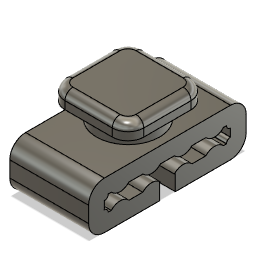
Helmet Mask Holder v3 (Autodesk Fusion 360 design; units mm, degrees)
Autodesk Fusion 360 part; units mm, degrees
sketch "Sketch1" plane through (0, 0, 0) normal (0, 1, 0) x (1, 0, 0)
  line L0 (-2770, 2200) -> (-2760, 2200)
  line L1 (-2760, 2200) -> (-2760, 2180)
  line L2 (-2760, 2180) -> (-2770, 2180)
  line L3 (-2770, 2180) -> (-2770, 2200)
  dimension "d3" = 10
  dimension "d4" = 20
  constraint horizontal L0
  constraint vertical L1
  constraint horizontal L2
  constraint vertical L3
  measures "d3" distance of L0.start L0.end
  measures "d4" distance of L0.start L2.end
extrude "Extrude1" add sketch "Sketch1" along normal blind 6 makes body 1
fillet "Fillet1" radius 2 4 edges at (-2765, 0, -2200) (-2765, 6, -2200) (-2765, 6, -2180) (-2765, 0, -2180) on bodies 1
sketch "Sketch2" plane through (-2760, 0, 0) normal (1, 0, 0) x (0, 0, -1)
  arc A0 (2180, 2) -> (2182, 0) centre (2182, 2) ccw
  line L0 (2182, 0) -> (2198, 0)
  arc A1 (2198, 0) -> (2200, 2) centre (2198, 2) ccw
  line L1 (2200, 2) -> (2200, 4)
  arc A2 (2200, 4) -> (2198, 6) centre (2198, 4) ccw
  line L2 (2198, 6) -> (2182, 6)
  arc A3 (2182, 6) -> (2180, 4) centre (2182, 4) ccw
  line L3 (2180, 4) -> (2180, 2)
  line L4 (2182, 4) -> (2198, 4)
  line L5 (2198, 4) -> (2198, 2)
  line L6 (2198, 2) -> (2182, 2)
  line L7 (2182, 2) -> (2182, 4)
  line L8 (2189.0127, 2) -> (2191, 2)
  line L9 (2191, 2) -> (2191, 0)
  line L10 (2191, 0) -> (2189.0127, 0)
  line L11 (2189.0127, 0) -> (2189.0127, 2)
  circle A4 centre (2184, 5) radius 1.5
  circle A5 centre (2184, 1) radius 1.5
  circle A6 centre (2188, 5) radius 1.5
  circle A7 centre (2188, 1) radius 1.5
  circle A8 centre (2192, 5) radius 1.5
  circle A9 centre (2192, 1) radius 1.5
  circle A10 centre (2196, 5) radius 1.5
  circle A11 centre (2196, 1) radius 1.5
  circle A12 centre (2182, 4) radius 0.5
  circle A13 centre (2182, 2) radius 0.5
  circle A14 centre (2198, 4) radius 0.5
  circle A15 centre (2198, 2) radius 0.5
  dimension "d9" = 3
  dimension "d10" = 3
  dimension "d11" = 3
  dimension "d12" = 3
  dimension "d13" = 3
  dimension "d14" = 3
  dimension "d15" = 3
  dimension "d16" = 3
  dimension "d28" = 1
  dimension "d29" = 1
  dimension "d30" = 1
  dimension "d31" = 1
  constraint horizontal L4
  constraint vertical L5
  constraint horizontal L6
  constraint vertical L7
  constraint coincident A1.centre L5.end
  constraint coincident A3.centre L4.start
  constraint horizontal L8
  constraint vertical L9
  constraint horizontal L10
  constraint vertical L11
  constraint coincident L0 L9.end
  constraint coincident L6 L8.start
  constraint concentric A0 A13
  constraint concentric A2 A14
  measures "d9" diameter of A4
  measures "d10" diameter of A5
  measures "d11" diameter of A6
  measures "d12" diameter of A7
  measures "d13" diameter of A8
  measures "d14" diameter of A9
  measures "d15" diameter of A10
  measures "d16" diameter of A11
  measures "d28" diameter of A12
  measures "d29" diameter of A13
  measures "d30" diameter of A14
  measures "d31" diameter of A15
extrude "Extrude2" cut sketch "Sketch2" against normal blind 30 contours L4 L5 L6 L7 L8 A4 A5 A6 A7 A8 A9 A10 A11 A12 A13 A14 A15 | L0 L6 L8 L10 L11 A7 | L0 L6 L8 L10 A7 A9 | L0 L6 L8 L9 L10 A9 bodies 1
sketch "Sketch3" plane through (0, 6, 0) normal (0, 1, 0) x (-1, 0, 0)
  line L0 (2770, -2182) -> (2760, -2182)
  line L1 (2760, -2182) -> (2760, -2198)
  line L2 (2770, -2198) -> (2770, -2182)
  circle A0 centre (2765, -2190) radius 4
  line L3 (2760, -2198) -> (2770, -2198)
  dimension "d27" = 8
  measures "d27" diameter of A0
extrude "Extrude3" add sketch "Sketch3" along normal blind 2 separate body contours A0 makes body 2
sketch "Sketch4" plane through (0, 8, 0) normal (0, 1, 0) x (-1, 0, 0)
  circle A0 centre (2765, -2190) radius 5
  circle A1 centre (2765, -2190) radius 4
  line L0 (2770, -2195) -> (2760, -2195)
  line L1 (2760, -2195) -> (2760, -2185)
  line L2 (2760, -2185) -> (2770, -2185)
  line L3 (2770, -2185) -> (2770, -2195)
  dimension "d21" = 10
  constraint horizontal L0
  constraint vertical L1
  constraint horizontal L2
  constraint vertical L3
  measures "d21" diameter of A0
extrude "Extrude4" add sketch "Sketch4" along normal blind 2 contours A0 | A0 L0 L3 | A0 L2 L3 | A0 L1 L2 | A0 L0 L1 | A1 bodies 1 2
fillet "Fillet2" [no effect]
combine "Combine1" operation add target body 1 tool bodies 2
fillet "Fillet3" radius 2 4 edges at (-2760, 9, -2185) (-2760, 9, -2195) (-2770, 9, -2185) (-2770, 9, -2195) on bodies 1
fillet "Fillet4" radius 1 8 edges at (-2769.4143, 10, -2194.4142) (-2770, 10, -2190) (-2769.4143, 10, -2185.5858) (-2765, 10, -2185) (-2760.5858, 10, -2185.5858) (-2760, 10, -2190) (-2760.5858, 10, -2194.4142) (-2765, 10, -2195) on bodies 1
